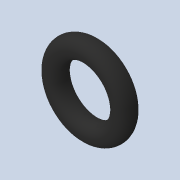
# Autodesk Inventor part: RollerTire
Saved by Autodesk Inventor 2020.4 (Build 244396000, 396)
## iProperties
Created: 2018-10-16
Part Number: RollerTire
Material: Rubber
Document SubType Name: Modeling
Designer: victo
Mass: 0.0511717 g
Surface Area: 1.06841 cm^2
Volume: 0.0550233 cm^3
Density: 0.93 g/cm^3
Appearance: Rubber - Black
Author: victo
Autodesk Inventor part; units mm, degrees
ref_plane "YZ Plane" through (0, 0, 0) normal (1, 0, 0) x (0, 1, 0)
ref_plane "XZ Plane" through (0, 0, 0) normal (0, 1, 0) x (-1, 0, 0)
ref_plane "XY Plane" through (0, 0, 0) normal (0, 0, 1) x (1, 0, 0)
sketch "Sketch1" plane through (0, 0, 0) normal (0, 0, 1) x (1, 0, 0)
  circle A0 centre (0, 0) radius 2.6275
  dimension "d0" = 5.255
  constraints: 1 centre point, 1 coincident
  measures "d0" diameter of A0
sketch "Sketch2" plane through (0, 0, 0) normal (0, 1, 0) x (-1, 0, 0)
  circle A0 centre (-3.6, 0) radius 1.05
  point P0 (0, 0)
  dimension "d1" = 2.1
  dimension "d2" = 3.6
  constraints: 1 centre point
  measures "d1" diameter of A0
  measures "d2" distance of point (0, 0) A0.centre
sweep "Tire Base" add profiles "Sketch2" path "Sketch1"
body "Solid1"
